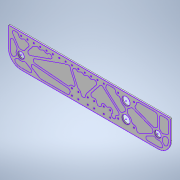
# Autodesk Inventor part: Part2
Saved by Autodesk Inventor 2021 (Build 250183000, 183)
## iProperties
Created: 2020-08-27
Part Number: Part2
Material: Generic
Document SubType Name: Modeling
Designer: gfellows
Density: 1 g/cm^3
Appearance: Default
Author: gfellows
Autodesk Inventor part; units mm, degrees
ref_plane "YZ Plane" through (0, 0, 0) normal (1, 0, 0) x (0, 1, 0)
ref_plane "XZ Plane" through (0, 0, 0) normal (0, 1, 0) x (-1, 0, 0)
ref_plane "XY Plane" through (0, 0, 0) normal (0, 0, 1) x (1, 0, 0)
sketch "Sketch2" plane through (0, 0, 0) normal (0, 0, 1) x (1, 0, 0)
  circle A0 centre (0, 0) radius 50 construction
  circle A1 centre (344, 0) radius 50 construction
  circle A2 centre (264, -8) radius 16 construction
  circle A3 centre (264, 32) radius 16 construction
  circle A4 centre (344, 0) radius 18.8 construction
  circle A5 centre (264, -8) radius 10 construction
  line L0 (261.9218, 1.7817) -> (340.093, 18.3896) construction
  line L1 (263.8999, -17.9995) -> (343.8119, -18.7991) construction
  circle A6 centre (264, 32) radius 10 construction
  circle A7 centre (0, 0) radius 18.8 construction
  line L2 (-1.6434, 18.728) -> (263.1259, 41.9617) construction
  line L3 (2.8786, -18.5783) -> (265.5312, 22.1179) construction
  arc A8 (-32, 0) -> (0, -32) centre (0, 0) ccw
  line L4 (0, -32) -> (344, -32)
  arc A9 (344, -32) -> (376, 0) centre (344, 0) ccw
  line L5 (-32, 0) -> (-32, 50)
  line L6 (-32, 50) -> (376, 50)
  line L7 (376, 50) -> (376, 0)
  circle A10 centre (264, 32) radius 3
  circle A11 centre (264, -8) radius 3
  circle A12 centre (0, 0) radius 8
  circle A13 centre (344, 0) radius 8
  circle A14 centre (264, 32) radius 10
  circle A15 centre (264, -8) radius 10
  circle A16 centre (284, 40) radius 1.5
  circle A17 centre (244, 40) radius 1.5
  circle A18 centre (244, -16) radius 1.5
  circle A19 centre (284, -16) radius 1.5
  circle A20 centre (0, 42) radius 1.5
  circle A21 centre (16, 42) radius 1.5
  circle A22 centre (32, 42) radius 1.5
  circle A23 centre (48, 42) radius 1.5
  circle A24 centre (64, 42) radius 1.5
  circle A25 centre (80, 42) radius 1.5
  circle A26 centre (96, 42) radius 1.5
  circle A27 centre (112, 42) radius 1.5
  circle A28 centre (128, 42) radius 1.5
  circle A29 centre (144, 42) radius 1.5
  circle A30 centre (160, 42) radius 1.5
  circle A31 centre (176, 42) radius 1.5
  circle A32 centre (192, 42) radius 1.5
  circle A33 centre (208, 42) radius 1.5
  circle A34 centre (128, -8) radius 1.5
  circle A35 centre (144, -8) radius 1.5
  circle A36 centre (128, -24) radius 1.5
  circle A37 centre (144, -24) radius 1.5
  circle A38 centre (184, -8) radius 1.5
  circle A39 centre (184, -24) radius 1.5
  circle A40 centre (168, -24) radius 1.5
  circle A41 centre (168, -8) radius 1.5
  circle A42 centre (224, -8) radius 1.5
  circle A43 centre (224, -24) radius 1.5
  circle A44 centre (208, -24) radius 1.5
  circle A45 centre (208, -8) radius 1.5
  dimension "d16" = 100
  dimension "d17" = 100
  dimension "d18" = 32
  dimension "d19" = 32
  dimension "d20" = 20
  dimension "d21" = 20
  dimension "d22" = 37.6
  dimension "d23" = 37.6
  dimension "d25" = 344
  dimension "d26" = 80
  dimension "d27" = 8
  dimension "d28" = 40
  dimension "d29" = 32
  dimension "d30" = 32
  dimension "d31" = 32
  dimension "d32" = 50
  dimension "d33" = 6
  dimension "d34" = 6
  dimension "d35" = 16
  dimension "d36" = 16
  dimension "d37" = 40
  dimension "d38" = 40
  dimension "d39" = 20
  dimension "d40" = 8
  dimension "d41" = 8
  dimension "d42" = 3
  dimension "d43" = 3
  dimension "d44" = 3
  dimension "d45" = 3
  dimension "d48" = 3
  dimension "d49" = 0
  dimension "d50" = 8
  dimension "d53" = 16
  dimension "d59" = 3
  dimension "d60" = 3
  dimension "d61" = 3
  dimension "d62" = 3
  dimension "d63" = 16
  dimension "d64" = 16
  dimension "d65" = 8
  dimension "d66" = 128
  dimension "d69" = 40
  constraints: 46 centre point, 16 end point, 13 coincident, 12 point on circle, 10 tangent, 5 horizontal alignment, 4 vertical alignment, 3 horizontal, 2 concentric, 2 vertical, 1 perpendicular, 42 other
  measures "d16" diameter of A0
  measures "d17" diameter of A1
  measures "d18" diameter of A2
  measures "d19" diameter of A3
  measures "d20" diameter of A6
  measures "d21" diameter of A5
  measures "d22" diameter of A7
  measures "d23" diameter of A4
  measures "d25" distance of A1.centre point (0, 0)
  measures "d26" horizontal distance of A1.centre A2.centre
  measures "d27" vertical distance of A1.centre A2.centre
  measures "d28" distance of A2.centre A3.centre
  measures "d29" distance from line of L5 point (0, 0)
  measures "d30" distance from line of L7 A1.centre
  measures "d31" distance from line of L4 A1.centre
  measures "d32" distance from line of L6 point (0, 0)
  measures "d33" diameter of A10
  measures "d34" diameter of A11
  measures "d35" diameter of A12
  measures "d36" diameter of A13
  measures "d37" distance of A16.centre A17.centre
  measures "d38" distance of A19.centre A18.centre
  measures "d39" horizontal distance of A19.centre A2.centre
  measures "d40" vertical distance of A3.centre A16.centre
  measures "d41" vertical distance of A19.centre A2.centre
  measures "d42" diameter of A17
  measures "d43" diameter of A16
  measures "d44" diameter of A19
  measures "d45" diameter of A18
  measures "d48" diameter of A20
  measures "d49" horizontal distance of A20.centre point (0, 0)
  measures "d50" distance from line of L6 A20.centre
  measures "d53" distance of A20.centre A21.centre
  measures "d59" diameter of A34
  measures "d60" diameter of A35
  measures "d61" diameter of A36
  measures "d62" diameter of A37
  measures "d63" distance of A34.centre A36.centre
  measures "d64" distance of A35.centre A34.centre
  measures "d65" distance from line of L4 A37.centre
  measures "d66" horizontal distance of point (0, 0) A34.centre
  measures "d69" distance of A35.centre A38.centre
extrude "Extrusion1" add sketch "Sketch2" along normal blind 3.175 contours L5 L6 L7 A9 L4 A8
fillet "Fillet1" radius 2 2 edges at (376, 50, 1.5875) (-32, 50, 1.5875)
sketch "Sketch7" plane through (0, 0, 3.175) normal (0, 0, 1) x (1, 0, 0)
  line L0 (374.4783, -9.6992) -> (375.5585, -5.1986)
  line L1 (375.5585, -5.1986) -> (375.6195, -4.8119)
  line L2 (375.6195, -4.8119) -> (375.9901, -0.0994)
  line L3 (375.9901, -0.0994) -> (376.0017, 0.0868)
  line L4 (376.0017, 0.0868) -> (376.0021, 47.8882)
  line L5 (376.0021, 47.8882) -> (375.9918, 48.0939)
  line L6 (375.9918, 48.0939) -> (375.9908, 48.1129)
  line L7 (375.9908, 48.1129) -> (375.9357, 48.4607)
  line L8 (375.9357, 48.4607) -> (375.8388, 48.7576)
  line L9 (375.8388, 48.7576) -> (375.6969, 49.0362)
  line L10 (375.6969, 49.0362) -> (375.514, 49.289)
  line L11 (375.514, 49.289) -> (375.2931, 49.5098)
  line L12 (375.2931, 49.5098) -> (375.0401, 49.6936)
  line L13 (375.0401, 49.6936) -> (374.7621, 49.8354)
  line L14 (374.7621, 49.8354) -> (374.4651, 49.9319)
  line L15 (374.4651, 49.9319) -> (374.1172, 49.987)
  line L16 (374.1172, 49.987) -> (374.0982, 49.9885)
  line L17 (374.0982, 49.9885) -> (373.9022, 49.9962)
  line L18 (373.9022, 49.9962) -> (-29.9016, 49.9999)
  line L19 (-29.9016, 49.9999) -> (-30.0978, 49.9922)
  line L20 (-30.0978, 49.9922) -> (-30.1168, 49.9907)
  line L21 (-30.1168, 49.9907) -> (-30.4647, 49.9356)
  line L22 (-30.4647, 49.9356) -> (-30.7616, 49.8392)
  line L23 (-30.7616, 49.8392) -> (-31.0401, 49.6974)
  line L24 (-31.0401, 49.6974) -> (-31.2929, 49.5138)
  line L25 (-31.2929, 49.5138) -> (-31.5136, 49.293)
  line L26 (-31.5136, 49.293) -> (-31.6972, 49.0402)
  line L27 (-31.6972, 49.0402) -> (-31.839, 48.7617)
  line L28 (-31.839, 48.7617) -> (-31.9355, 48.4648)
  line L29 (-31.9355, 48.4648) -> (-31.9906, 48.117)
  line L30 (-31.9906, 48.117) -> (-31.9921, 48.098)
  line L31 (-31.9921, 48.098) -> (-31.9998, 47.9018)
  line L32 (-31.9998, 47.9018) -> (-32.0002, 0.098)
  line L33 (-32.0002, 0.098) -> (-31.9925, -0.0977)
  line L34 (-31.9925, -0.0977) -> (-31.6216, -4.8101)
  line L35 (-31.6216, -4.8101) -> (-31.5604, -5.1969)
  line L36 (-31.5604, -5.1969) -> (-30.4798, -9.6975)
  line L37 (-30.4798, -9.6975) -> (-30.3588, -10.07)
  line L38 (-30.3588, -10.07) -> (-28.5887, -14.3466)
  line L39 (-28.5887, -14.3466) -> (-28.4108, -14.6956)
  line L40 (-28.4108, -14.6956) -> (-25.9924, -18.642)
  line L41 (-25.9924, -18.642) -> (-25.7621, -18.9589)
  line L42 (-25.7621, -18.9589) -> (-22.7562, -22.4784)
  line L43 (-22.7562, -22.4784) -> (-22.4791, -22.7554)
  line L44 (-22.4791, -22.7554) -> (-18.9589, -25.7604)
  line L45 (-18.9589, -25.7604) -> (-18.642, -25.9907)
  line L46 (-18.642, -25.9907) -> (-14.6957, -28.4092)
  line L47 (-14.6957, -28.4092) -> (-14.3467, -28.587)
  line L48 (-14.3467, -28.587) -> (-10.0704, -30.3582)
  line L49 (-10.0704, -30.3582) -> (-9.698, -30.4792)
  line L50 (-9.698, -30.4792) -> (-5.1972, -31.5594)
  line L51 (-5.1972, -31.5594) -> (-4.8105, -31.6206)
  line L52 (-4.8105, -31.6206) -> (-0.098, -31.9913)
  line L53 (-0.098, -31.9913) -> (0.0977, -31.9989)
  line L54 (0.0977, -31.9989) -> (343.9017, -32.0021)
  line L55 (343.9017, -32.0021) -> (344.0977, -31.9944)
  line L56 (344.0977, -31.9944) -> (348.8097, -31.6235)
  line L57 (348.8097, -31.6235) -> (349.1967, -31.5622)
  line L58 (349.1967, -31.5622) -> (353.6976, -30.4816)
  line L59 (353.6976, -30.4816) -> (354.0696, -30.3606)
  line L60 (354.0696, -30.3606) -> (358.3461, -28.5905)
  line L61 (358.3461, -28.5905) -> (358.6951, -28.4127)
  line L62 (358.6951, -28.4127) -> (362.6419, -25.9939)
  line L63 (362.6419, -25.9939) -> (362.9589, -25.7636)
  line L64 (362.9589, -25.7636) -> (366.4781, -22.758)
  line L65 (366.4781, -22.758) -> (366.755, -22.4809)
  line L66 (366.755, -22.4809) -> (369.7602, -18.9606)
  line L67 (369.7602, -18.9606) -> (369.9901, -18.6437)
  line L68 (369.9901, -18.6437) -> (372.4087, -14.6971)
  line L69 (372.4087, -14.6971) -> (372.5857, -14.3481)
  line L70 (372.5857, -14.3481) -> (374.3573, -10.0717)
  line L71 (374.3573, -10.0717) -> (374.4783, -9.6992)
  line L72 (353.5083, 8.3734) -> (350.2762, 10.7218)
  line L73 (350.2762, 10.7218) -> (348.4596, 13.2222)
  line L74 (348.4596, 13.2222) -> (348.2149, 14.7673)
  line L75 (348.2149, 14.7673) -> (348.2151, 40)
  line L76 (348.2151, 40) -> (349.1701, 42.9389)
  line L77 (349.1701, 42.9389) -> (353.2152, 44.9998)
  line L78 (353.2152, 44.9998) -> (366.0002, 44.9997)
  line L79 (366.0002, 44.9997) -> (368.9391, 44.0447)
  line L80 (368.9391, 44.0447) -> (370.9989, 40.0018)
  line L81 (370.9989, 40.0018) -> (370.9987, 15.8213)
  line L82 (370.9987, 15.8213) -> (370.0438, 12.8824)
  line L83 (370.0438, 12.8824) -> (367.6762, 11.1097)
  line L84 (367.6762, 11.1097) -> (358.1243, 7.7084)
  line L85 (358.1243, 7.7084) -> (355.0353, 7.6221)
  line L86 (355.0353, 7.6221) -> (353.5083, 8.3734)
  line L87 (-2.3107, 12.3636) -> (-5.2496, 13.3185)
  line L88 (-5.2496, 13.3185) -> (-6.5079, 14.6465)
  line L89 (-6.5079, 14.6465) -> (-21.1616, 37.2829)
  line L90 (-21.1616, 37.2829) -> (-21.9571, 40.2689)
  line L91 (-21.9571, 40.2689) -> (-20.8455, 43.1522)
  line L92 (-20.8455, 43.1522) -> (-16.9643, 44.9999)
  line L93 (-16.9643, 44.9999) -> (-11.1074, 44.9999)
  line L94 (-11.1074, 44.9999) -> (-8.1685, 44.0449)
  line L95 (-8.1685, 44.0449) -> (-6.3521, 41.5449)
  line L96 (-6.3521, 41.5449) -> (-5.5034, 38.9323)
  line L97 (-5.5034, 38.9323) -> (-4.618, 37.7137)
  line L98 (-4.618, 37.7137) -> (-2.6494, 36.2833)
  line L99 (-2.6494, 36.2833) -> (-1.2168, 35.8178)
  line L100 (-1.2168, 35.8178) -> (1.2166, 35.8178)
  line L101 (1.2166, 35.8178) -> (2.6492, 36.2832)
  line L102 (2.6492, 36.2832) -> (5.061, 38.0355)
  line L103 (5.061, 38.0355) -> (8, 38.9903)
  line L104 (8, 38.9903) -> (10.9389, 38.0353)
  line L105 (10.9389, 38.0353) -> (13.3507, 36.2829)
  line L106 (13.3507, 36.2829) -> (15.5364, 35.5727)
  line L107 (15.5364, 35.5727) -> (15.5209, 35.5249)
  line L108 (15.5209, 35.5249) -> (17.558, 34.863)
  line L109 (17.558, 34.863) -> (19.3743, 32.363)
  line L110 (19.3743, 32.363) -> (19.3743, 29.2728)
  line L111 (19.3743, 29.2728) -> (18.5549, 27.7343)
  line L112 (18.5549, 27.7343) -> (8.0015, 14.2642)
  line L113 (8.0015, 14.2642) -> (5.4373, 12.5397)
  line L114 (5.4373, 12.5397) -> (4.0171, 12.5655)
  line L115 (4.0171, 12.5655) -> (4.0171, 12.3635)
  line L116 (4.0171, 12.3635) -> (-2.3107, 12.3636)
  line L117 (331.309, 10.0791) -> (331.29, 10.0442)
  line L118 (331.29, 10.0442) -> (331.108, 10.1445)
  line L119 (331.108, 10.1445) -> (331.068, 10.1573)
  line L120 (331.068, 10.1573) -> (331.017, 10.1946)
  line L121 (331.017, 10.1946) -> (330.476, 10.493)
  line L122 (330.476, 10.493) -> (289.462, 26.8484)
  line L123 (289.462, 26.8484) -> (287.086, 28.824)
  line L124 (287.086, 28.824) -> (286.325, 31.819)
  line L125 (286.325, 31.819) -> (288.376, 35.5378)
  line L126 (288.376, 35.5378) -> (288.618, 35.7139)
  line L127 (288.618, 35.7139) -> (289.5033, 36.9323)
  line L128 (289.5033, 36.9323) -> (290.2553, 39.2466)
  line L129 (290.2553, 39.2466) -> (290.2553, 39.9998)
  line L130 (290.2553, 39.9998) -> (291.2102, 42.9387)
  line L131 (291.2102, 42.9387) -> (295.2553, 44.9996)
  line L132 (295.2553, 44.9996) -> (338.2153, 44.9992)
  line L133 (338.2153, 44.9992) -> (341.1543, 44.0442)
  line L134 (341.1543, 44.0442) -> (343.2152, 39.9991)
  line L135 (343.2152, 39.9991) -> (343.215, 16.7886)
  line L136 (343.215, 16.7886) -> (342.2612, 13.8504)
  line L137 (342.2612, 13.8504) -> (339.7612, 12.034)
  line L138 (339.7612, 12.034) -> (339.3422, 11.8981)
  line L139 (339.3422, 11.8981) -> (336.9461, 10.1573)
  line L140 (336.9461, 10.1573) -> (334.007, 9.2025)
  line L141 (334.007, 9.2025) -> (331.309, 10.0791)
  line L142 (247.7696, 2.7223) -> (214.4517, 32.6032)
  line L143 (214.4517, 32.6032) -> (212.901, 35.2763)
  line L144 (212.901, 35.2763) -> (213.499, 38.1013)
  line L145 (213.499, 38.1013) -> (213.259, 38.1794)
  line L146 (213.259, 38.1794) -> (214.3526, 41.5449)
  line L147 (214.3526, 41.5449) -> (216.1692, 44.0452)
  line L148 (216.1692, 44.0452) -> (219.1073, 44.9997)
  line L149 (219.1073, 44.9997) -> (232.7453, 44.9995)
  line L150 (232.7453, 44.9995) -> (235.6843, 44.0446)
  line L151 (235.6843, 44.0446) -> (237.7453, 39.9994)
  line L152 (237.7453, 39.9994) -> (237.7452, 39.2463)
  line L153 (237.7452, 39.2463) -> (238.4971, 36.9319)
  line L154 (238.4971, 36.9319) -> (239.3824, 35.7135)
  line L155 (239.3824, 35.7135) -> (241.3512, 34.2829)
  line L156 (241.3512, 34.2829) -> (242.7832, 33.8176)
  line L157 (242.7832, 33.8176) -> (244.7772, 33.8176)
  line L158 (244.7772, 33.8176) -> (247.7153, 32.8629)
  line L159 (247.7153, 32.8629) -> (249.5319, 30.3626)
  line L160 (249.5319, 30.3626) -> (251.6197, 23.9358)
  line L161 (251.6197, 23.9358) -> (252.505, 22.7173)
  line L162 (252.505, 22.7173) -> (259.3646, 17.7331)
  line L163 (259.3646, 17.7331) -> (259.3596, 17.7292)
  line L164 (259.3596, 17.7292) -> (261.2138, 16.3819)
  line L165 (261.2138, 16.3819) -> (262.1688, 13.4423)
  line L166 (262.1688, 13.4423) -> (262.1688, 10.5493)
  line L167 (262.1688, 10.5493) -> (261.2138, 7.6103)
  line L168 (261.2138, 7.6103) -> (259.3599, 6.2634)
  line L169 (259.3599, 6.2634) -> (259.3602, 6.2608)
  line L170 (259.3602, 6.2608) -> (254.0454, 2.3993)
  line L171 (254.0454, 2.3993) -> (251.1064, 1.4445)
  line L172 (251.1064, 1.4445) -> (247.7696, 2.7223)
  line L173 (17.8113, 12.6027) -> (16.7825, 15.5166)
  line L174 (16.7825, 15.5166) -> (17.845, 18.7263)
  line L175 (17.845, 18.7263) -> (29.7343, 33.9016)
  line L176 (29.7343, 33.9016) -> (32.5598, 35.2774)
  line L177 (32.5598, 35.2774) -> (32.4631, 35.5753)
  line L178 (32.4631, 35.5753) -> (34.6488, 36.2854)
  line L179 (34.6488, 36.2854) -> (37.0606, 38.0376)
  line L180 (37.0606, 38.0376) -> (39.9995, 38.9924)
  line L181 (39.9995, 38.9924) -> (42.9384, 38.0375)
  line L182 (42.9384, 38.0375) -> (45.3502, 36.2851)
  line L183 (45.3502, 36.2851) -> (46.7827, 35.8196)
  line L184 (46.7827, 35.8196) -> (49.2161, 35.8196)
  line L185 (49.2161, 35.8196) -> (50.6488, 36.285)
  line L186 (50.6488, 36.285) -> (53.0606, 38.0373)
  line L187 (53.0606, 38.0373) -> (55.9995, 38.992)
  line L188 (55.9995, 38.992) -> (58.9384, 38.0371)
  line L189 (58.9384, 38.0371) -> (61.3502, 36.2847)
  line L190 (61.3502, 36.2847) -> (62.7827, 35.8192)
  line L191 (62.7827, 35.8192) -> (64.7633, 35.8192)
  line L192 (64.7633, 35.8192) -> (66.1505, 35.3685)
  line L193 (66.1505, 35.3685) -> (66.227, 35.6258)
  line L194 (66.227, 35.6258) -> (67.406, 36.8349)
  line L195 (67.406, 36.8349) -> (69.0605, 38.037)
  line L196 (69.0605, 38.037) -> (71.9995, 38.9917)
  line L197 (71.9995, 38.9917) -> (74.9384, 38.0368)
  line L198 (74.9384, 38.0368) -> (75.5107, 37.6209)
  line L199 (75.5107, 37.6209) -> (77.3273, 35.1206)
  line L200 (77.3273, 35.1206) -> (77.3273, 32.0304)
  line L201 (77.3273, 32.0304) -> (74.2367, 28.8607)
  line L202 (74.2367, 28.8607) -> (72.0099, 28.0745)
  line L203 (72.0099, 28.0745) -> (68.9207, 27.9965)
  line L204 (68.9207, 27.9965) -> (68.5337, 28.263)
  line L205 (68.5337, 28.263) -> (66.4283, 26.1038)
  line L206 (66.4283, 26.1038) -> (23.4455, 10.928)
  line L207 (23.4455, 10.928) -> (20.3563, 10.85)
  line L208 (20.3563, 10.85) -> (17.8113, 12.6027)
  line L209 (155.2548, -13.6224) -> (152.3158, -12.6675)
  line L210 (152.3158, -12.6675) -> (150.2549, -8.6224)
  line L211 (150.2549, -8.6224) -> (150.255, -7.2468)
  line L212 (150.255, -7.2468) -> (149.5031, -4.9325)
  line L213 (149.5031, -4.9325) -> (148.6179, -3.7141)
  line L214 (148.6179, -3.7141) -> (146.649, -2.2835)
  line L215 (146.649, -2.2835) -> (145.592, -1.9401)
  line L216 (145.592, -1.9401) -> (142.543, 0.8412)
  line L217 (142.543, 0.8412) -> (129.684, 30.7658)
  line L218 (129.684, 30.7658) -> (129.401, 33.843)
  line L219 (129.401, 33.843) -> (131.339, 36.7849)
  line L220 (131.339, 36.7849) -> (133.0609, 38.036)
  line L221 (133.0609, 38.036) -> (136, 38.9908)
  line L222 (136, 38.9908) -> (138.939, 38.0358)
  line L223 (138.939, 38.0358) -> (141.3509, 36.2833)
  line L224 (141.3509, 36.2833) -> (142.7829, 35.818)
  line L225 (142.7829, 35.818) -> (145.2169, 35.818)
  line L226 (145.2169, 35.818) -> (146.649, 36.2832)
  line L227 (146.649, 36.2832) -> (149.0609, 38.0356)
  line L228 (149.0609, 38.0356) -> (152, 38.9904)
  line L229 (152, 38.9904) -> (154.939, 38.0354)
  line L230 (154.939, 38.0354) -> (157.3508, 36.283)
  line L231 (157.3508, 36.283) -> (158.7829, 35.8177)
  line L232 (158.7829, 35.8177) -> (161.2169, 35.8176)
  line L233 (161.2169, 35.8176) -> (162.649, 36.2829)
  line L234 (162.649, 36.2829) -> (165.0609, 38.0352)
  line L235 (165.0609, 38.0352) -> (168, 38.99)
  line L236 (168, 38.99) -> (170.939, 38.0351)
  line L237 (170.939, 38.0351) -> (173.3508, 36.2826)
  line L238 (173.3508, 36.2826) -> (174.7829, 35.8173)
  line L239 (174.7829, 35.8173) -> (177.2169, 35.8173)
  line L240 (177.2169, 35.8173) -> (178.649, 36.2825)
  line L241 (178.649, 36.2825) -> (181.0609, 38.0349)
  line L242 (181.0609, 38.0349) -> (184, 38.9897)
  line L243 (184, 38.9897) -> (186.9389, 38.0347)
  line L244 (186.9389, 38.0347) -> (188.324, 37.0283)
  line L245 (188.324, 37.0283) -> (190.1406, 34.528)
  line L246 (190.1406, 34.528) -> (190.1406, 31.4378)
  line L247 (190.1406, 31.4378) -> (189.2972, 29.861)
  line L248 (189.2972, 29.861) -> (164.7591, -0.8634)
  line L249 (164.7591, -0.8634) -> (164.338, -1.6443)
  line L250 (164.338, -1.6443) -> (164.1399, -2.2549)
  line L251 (164.1399, -2.2549) -> (163.4297, -3.6487)
  line L252 (163.4297, -3.6487) -> (162.4968, -4.9327)
  line L253 (162.4968, -4.9327) -> (161.7448, -7.247)
  line L254 (161.7448, -7.247) -> (161.7448, -8.6225)
  line L255 (161.7448, -8.6225) -> (160.7899, -11.5614)
  line L256 (160.7899, -11.5614) -> (158.2898, -13.3777)
  line L257 (158.2898, -13.3777) -> (156.7448, -13.6224)
  line L258 (156.7448, -13.6224) -> (155.2548, -13.6224)
  line L259 (34.6019, -0.5648) -> (31.7567, 0.6412)
  line L260 (31.7567, 0.6412) -> (30.1637, 3.2891)
  line L261 (30.1637, 3.2891) -> (30.4315, 6.3677)
  line L262 (30.4315, 6.3677) -> (33.3706, 9.131)
  line L263 (33.3706, 9.131) -> (104.1632, 34.1255)
  line L264 (104.1632, 34.1255) -> (104.7972, 34.4586)
  line L265 (104.7972, 34.4586) -> (105.7552, 35.1541)
  line L266 (105.7552, 35.1541) -> (105.8754, 34.9886)
  line L267 (105.8754, 34.9886) -> (107.2256, 35.9695)
  line L268 (107.2256, 35.9695) -> (110.3166, 35.9695)
  line L269 (110.3166, 35.9695) -> (110.7836, 35.8175)
  line L270 (110.7836, 35.8175) -> (113.2176, 35.8175)
  line L271 (113.2176, 35.8175) -> (114.6497, 36.2828)
  line L272 (114.6497, 36.2828) -> (116.3065, 37.4865)
  line L273 (116.3065, 37.4865) -> (119.2455, 38.4413)
  line L274 (119.2455, 38.4413) -> (122.1845, 37.4863)
  line L275 (122.1845, 37.4863) -> (124.2454, 33.4412)
  line L276 (124.2454, 33.4412) -> (124.2454, 31.2461)
  line L277 (124.2454, 31.2461) -> (124.4423, 30.6389)
  line L278 (124.4423, 30.6389) -> (124.5233, 30.4242)
  line L279 (124.5233, 30.4242) -> (135.5081, 4.8609)
  line L280 (135.5081, 4.8609) -> (135.7911, 1.7846)
  line L281 (135.7911, 1.7846) -> (134.2113, -0.8714)
  line L282 (134.2113, -0.8714) -> (131.3723, -2.0914)
  line L283 (131.3723, -2.0914) -> (129.3693, -1.8677)
  line L284 (129.3693, -1.8677) -> (129.2173, -1.8183)
  line L285 (129.2173, -1.8183) -> (126.7833, -1.8182)
  line L286 (126.7833, -1.8182) -> (125.3513, -2.2835)
  line L287 (125.3513, -2.2835) -> (123.3824, -3.7139)
  line L288 (123.3824, -3.7139) -> (122.0295, -5.5759)
  line L289 (122.0295, -5.5759) -> (121.8738, -5.4628)
  line L290 (121.8738, -5.4628) -> (120.8734, -6.8396)
  line L291 (120.8734, -6.8396) -> (117.5014, -7.7756)
  line L292 (117.5014, -7.7756) -> (34.6019, -0.5648)
  line L293 (228.6909, -19.8299) -> (228.1429, -19.0767)
  line L294 (228.1429, -19.0767) -> (228.2839, -18.9744)
  line L295 (228.2839, -18.9744) -> (227.248, -17.5486)
  line L296 (227.248, -17.5486) -> (227.2481, -14.4584)
  line L297 (227.2481, -14.4584) -> (228.2841, -13.0325)
  line L298 (228.2841, -13.0325) -> (228.1431, -12.9302)
  line L299 (228.1431, -12.9302) -> (228.6912, -12.1771)
  line L300 (228.6912, -12.1771) -> (230.8133, -10.6353)
  line L301 (230.8133, -10.6353) -> (230.2466, -8.891)
  line L302 (230.2466, -8.891) -> (230.2467, -7.2504)
  line L303 (230.2467, -7.2504) -> (229.4948, -4.936)
  line L304 (229.4948, -4.936) -> (228.6096, -3.7176)
  line L305 (228.6096, -3.7176) -> (226.6407, -2.2871)
  line L306 (226.6407, -2.2871) -> (225.2087, -1.8217)
  line L307 (225.2087, -1.8217) -> (222.7747, -1.8217)
  line L308 (222.7747, -1.8217) -> (221.3426, -2.2869)
  line L309 (221.3426, -2.2869) -> (218.9307, -4.0393)
  line L310 (218.9307, -4.0393) -> (215.9916, -4.9941)
  line L311 (215.9916, -4.9941) -> (213.0526, -4.0391)
  line L312 (213.0526, -4.0391) -> (210.6408, -2.2867)
  line L313 (210.6408, -2.2867) -> (209.2087, -1.8214)
  line L314 (209.2087, -1.8214) -> (206.7747, -1.8214)
  line L315 (206.7747, -1.8214) -> (205.3426, -2.2866)
  line L316 (205.3426, -2.2866) -> (203.3738, -3.7171)
  line L317 (203.3738, -3.7171) -> (202.4885, -4.9355)
  line L318 (202.4885, -4.9355) -> (201.7365, -7.2498)
  line L319 (201.7365, -7.2498) -> (201.7365, -8.6253)
  line L320 (201.7365, -8.6253) -> (200.7815, -11.5642)
  line L321 (200.7815, -11.5642) -> (198.2815, -13.3805)
  line L322 (198.2815, -13.3805) -> (196.7365, -13.6252)
  line L323 (196.7365, -13.6252) -> (195.2465, -13.6252)
  line L324 (195.2465, -13.6252) -> (192.3075, -12.6703)
  line L325 (192.3075, -12.6703) -> (190.2466, -8.6252)
  line L326 (190.2466, -8.6252) -> (190.2466, -7.2496)
  line L327 (190.2466, -7.2496) -> (189.4948, -4.9353)
  line L328 (189.4948, -4.9353) -> (188.6095, -3.7169)
  line L329 (188.6095, -3.7169) -> (186.6407, -2.2863)
  line L330 (186.6407, -2.2863) -> (185.2087, -1.821)
  line L331 (185.2087, -1.821) -> (182.7747, -1.821)
  line L332 (182.7747, -1.821) -> (181.8897, -2.1085)
  line L333 (181.8897, -2.1085) -> (178.7997, -2.1085)
  line L334 (178.7997, -2.1085) -> (176.2997, -0.292)
  line L335 (176.2997, -0.292) -> (175.3449, 2.647)
  line L336 (175.3449, 2.647) -> (176.4382, 5.7666)
  line L337 (176.4382, 5.7666) -> (198.4957, 33.3851)
  line L338 (198.4957, 33.3851) -> (201.0759, 35.0857)
  line L339 (201.0759, 35.0857) -> (204.1629, 34.9448)
  line L340 (204.1629, 34.9448) -> (205.9007, 33.5484)
  line L341 (205.9007, 33.5484) -> (205.9727, 33.6296)
  line L342 (205.9727, 33.6296) -> (244.8683, -1.2536)
  line L343 (244.8683, -1.2536) -> (246.419, -3.9267)
  line L344 (246.419, -3.9267) -> (246.1032, -6.9928)
  line L345 (246.1032, -6.9928) -> (243.0761, -9.7238)
  line L346 (243.0761, -9.7238) -> (241.342, -10.2871)
  line L347 (241.342, -10.2871) -> (239.3732, -11.7176)
  line L348 (239.3732, -11.7176) -> (239.2912, -11.8301)
  line L349 (239.2912, -11.8301) -> (237.1691, -13.3719)
  line L350 (237.1691, -13.3719) -> (237.7357, -15.1162)
  line L351 (237.7357, -15.1162) -> (237.7357, -16.8911)
  line L352 (237.7357, -16.8911) -> (236.7808, -19.83)
  line L353 (236.7808, -19.83) -> (234.2808, -21.6464)
  line L354 (234.2808, -21.6464) -> (231.1908, -21.6464)
  line L355 (231.1908, -21.6464) -> (228.6909, -19.8299)
  line L356 (-23.26, -11.7395) -> (-25.216, -9.4204)
  line L357 (-25.216, -9.4204) -> (-25.5133, -8.7021)
  line L358 (-25.5133, -8.7021) -> (-25.7557, -7.956)
  line L359 (-25.7557, -7.956) -> (-26.5605, -4.604)
  line L360 (-26.5605, -4.604) -> (-26.6832, -3.8291)
  line L361 (-26.6832, -3.8291) -> (-26.9847, 0.0007)
  line L362 (-26.9847, 0.0007) -> (-27.0001, 0.393)
  line L363 (-27.0001, 0.393) -> (-26.9999, 20.1896)
  line L364 (-26.9999, 20.1896) -> (-26.045, 23.1285)
  line L365 (-26.045, 23.1285) -> (-23.545, 24.9449)
  line L366 (-23.545, 24.9449) -> (-20.4548, 24.9448)
  line L367 (-20.4548, 24.9448) -> (-17.8026, 22.9066)
  line L368 (-17.8026, 22.9066) -> (-10.866, 12.1912)
  line L369 (-10.866, 12.1912) -> (-10.0705, 9.2052)
  line L370 (-10.0705, 9.2052) -> (-10.6145, 7.6727)
  line L371 (-10.6145, 7.6727) -> (-10.5154, 7.6404)
  line L372 (-10.5154, 7.6404) -> (-12.7544, 0.7496)
  line L373 (-12.7544, 0.7496) -> (-12.7544, -0.7567)
  line L374 (-12.7544, -0.7567) -> (-12.0806, -2.8307)
  line L375 (-12.0806, -2.8307) -> (-12.0807, -5.9209)
  line L376 (-12.0807, -5.9209) -> (-13.6347, -8.2157)
  line L377 (-13.6347, -8.2157) -> (-17.3951, -11.3494)
  line L378 (-17.3951, -11.3494) -> (-20.2642, -12.4973)
  line L379 (-20.2642, -12.4973) -> (-23.26, -11.7395)
  line L380 (291.6642, -20.353) -> (290.2542, -16.8733)
  line L381 (290.2542, -16.8733) -> (290.2542, -15.2472)
  line L382 (290.2542, -15.2472) -> (289.5024, -12.9328)
  line L383 (289.5024, -12.9328) -> (288.6171, -11.7144)
  line L384 (288.6171, -11.7144) -> (286.6483, -10.2838)
  line L385 (286.6483, -10.2838) -> (285.2163, -9.8185)
  line L386 (285.2163, -9.8185) -> (283.2223, -9.8185)
  line L387 (283.2223, -9.8185) -> (280.2842, -8.8638)
  line L388 (280.2842, -8.8638) -> (278.4676, -6.3635)
  line L389 (278.4676, -6.3635) -> (276.3798, 0.0633)
  line L390 (276.3798, 0.0633) -> (275.4945, 1.2818)
  line L391 (275.4945, 1.2818) -> (269.2329, 5.8314)
  line L392 (269.2329, 5.8314) -> (267.4167, 8.3313)
  line L393 (267.4167, 8.3313) -> (267.172, 9.8764)
  line L394 (267.172, 9.8764) -> (267.172, 14.1236)
  line L395 (267.172, 14.1236) -> (268.127, 17.0625)
  line L396 (268.127, 17.0625) -> (269.2328, 18.1689)
  line L397 (269.2328, 18.1689) -> (275.4945, 22.7183)
  line L398 (275.4945, 22.7183) -> (275.6475, 22.9294)
  line L399 (275.6475, 22.9294) -> (278.1475, 24.7458)
  line L400 (278.1475, 24.7458) -> (281.5445, 24.6347)
  line L401 (281.5445, 24.6347) -> (328.0966, 6.0709)
  line L402 (328.0966, 6.0709) -> (330.4726, 4.0953)
  line L403 (330.4726, 4.0953) -> (331.2446, 1.4265)
  line L404 (331.2446, 1.4265) -> (331.2446, -1.5458)
  line L405 (331.2446, -1.5458) -> (331.0404, -1.5458)
  line L406 (331.0404, -1.5458) -> (331.0403, -3.2159)
  line L407 (331.0403, -3.2159) -> (328.4843, -6.1608)
  line L408 (328.4843, -6.1608) -> (297.4542, -21.3634)
  line L409 (297.4542, -21.3634) -> (294.3952, -21.7989)
  line L410 (294.3952, -21.7989) -> (291.6642, -20.353)
  line L411 (359.132, -14.5813) -> (356.029, -11.192)
  line L412 (356.029, -11.192) -> (354.749, -8.3794)
  line L413 (354.749, -8.3794) -> (354.962, -6.271)
  line L414 (354.962, -6.271) -> (356.975, -0.0757)
  line L415 (356.975, -0.0757) -> (360.0541, 3.0895)
  line L416 (360.0541, 3.0895) -> (364.283, 4.5954)
  line L417 (364.283, 4.5954) -> (367.372, 4.6817)
  line L418 (367.372, 4.6817) -> (369.9221, 2.9359)
  line L419 (369.9221, 2.9359) -> (370.9453, -0.5069)
  line L420 (370.9453, -0.5069) -> (370.6834, -3.829)
  line L421 (370.6834, -3.829) -> (370.5603, -4.6039)
  line L422 (370.5603, -4.6039) -> (369.7559, -7.9558)
  line L423 (369.7559, -7.9558) -> (369.5128, -8.7019)
  line L424 (369.5128, -8.7019) -> (368.1937, -11.8869)
  line L425 (368.1937, -11.8869) -> (367.8377, -12.586)
  line L426 (367.8377, -12.586) -> (367.0829, -13.8177)
  line L427 (367.0829, -13.8177) -> (364.733, -15.8247)
  line L428 (364.733, -15.8247) -> (361.653, -16.0672)
  line L429 (361.653, -16.0672) -> (359.132, -14.5813)
  line L430 (49.5735, -27.0002) -> (46.6346, -26.0453)
  line L431 (46.6346, -26.0453) -> (45.7411, -25.3961)
  line L432 (45.7411, -25.3961) -> (45.5849, -25.2914)
  line L433 (45.5849, -25.2914) -> (27.9029, -14.3736)
  line L434 (27.9029, -14.3736) -> (25.9039, -12.0171)
  line L435 (25.9039, -12.0171) -> (25.6718, -8.9357)
  line L436 (25.6718, -8.9357) -> (27.2953, -6.3063)
  line L437 (27.2953, -6.3063) -> (30.963, -5.138)
  line L438 (30.963, -5.138) -> (119.04, -12.7991)
  line L439 (119.04, -12.7991) -> (121.885, -14.0051)
  line L440 (121.885, -14.0051) -> (123.478, -16.653)
  line L441 (123.478, -16.653) -> (122.6516, -20.7201)
  line L442 (122.6516, -20.7201) -> (122.4966, -20.9335)
  line L443 (122.4966, -20.9335) -> (121.6477, -23.5461)
  line L444 (121.6477, -23.5461) -> (119.831, -26.0463)
  line L445 (119.831, -26.0463) -> (116.8929, -27.0008)
  line L446 (116.8929, -27.0008) -> (49.5735, -27.0002)
  line L447 (318.7702, -26.9999) -> (315.8312, -26.0449)
  line L448 (315.8312, -26.0449) -> (314.015, -23.5451)
  line L449 (314.015, -23.5451) -> (314.015, -20.4549)
  line L450 (314.015, -20.4549) -> (316.57, -17.5099)
  line L451 (316.57, -17.5099) -> (332.0801, -9.9111)
  line L452 (332.0801, -9.9111) -> (335.1401, -9.4755)
  line L453 (335.1401, -9.4755) -> (337.2191, -10.3559)
  line L454 (337.2191, -10.3559) -> (339.342, -11.8984)
  line L455 (339.342, -11.8984) -> (340.775, -12.364)
  line L456 (340.775, -12.364) -> (348.0185, -12.3641)
  line L457 (348.0185, -12.3641) -> (348.0185, -12.5721)
  line L458 (348.0185, -12.5721) -> (349.6772, -12.5721)
  line L459 (349.6772, -12.5721) -> (351.8202, -13.9516)
  line L460 (351.8202, -13.9516) -> (354.9182, -17.3363)
  line L461 (354.9182, -17.3363) -> (356.1982, -20.149)
  line L462 (356.1982, -20.149) -> (355.5807, -23.1767)
  line L463 (355.5807, -23.1767) -> (353.1433, -25.331)
  line L464 (353.1433, -25.331) -> (352.7022, -25.5133)
  line L465 (352.7022, -25.5133) -> (351.9562, -25.7557)
  line L466 (351.9562, -25.7557) -> (348.6042, -26.5605)
  line L467 (348.6042, -26.5605) -> (347.8292, -26.6832)
  line L468 (347.8292, -26.6832) -> (343.9992, -26.9847)
  line L469 (343.9992, -26.9847) -> (343.6072, -27.0001)
  line L470 (343.6072, -27.0001) -> (318.7702, -26.9999)
  line L471 (0.3931, -26.9995) -> (0.0007, -26.9841)
  line L472 (0.0007, -26.9841) -> (-3.829, -26.6829)
  line L473 (-3.829, -26.6829) -> (-4.604, -26.5601)
  line L474 (-4.604, -26.5601) -> (-7.956, -25.7557)
  line L475 (-7.956, -25.7557) -> (-8.7022, -25.5132)
  line L476 (-8.7022, -25.5132) -> (-11.8872, -24.194)
  line L477 (-11.8872, -24.194) -> (-12.5863, -23.8378)
  line L478 (-12.5863, -23.8378) -> (-13.6874, -23.163)
  line L479 (-13.6874, -23.163) -> (-15.6943, -20.8132)
  line L480 (-15.6943, -20.8132) -> (-15.9368, -17.7326)
  line L481 (-15.9368, -17.7326) -> (-14.2769, -15.0595)
  line L482 (-14.2769, -15.0595) -> (-10.7618, -12.1303)
  line L483 (-10.7618, -12.1303) -> (-7.8927, -10.9824)
  line L484 (-7.8927, -10.9824) -> (-5.4231, -11.6954)
  line L485 (-5.4231, -11.6954) -> (-5.4099, -11.6548)
  line L486 (-5.4099, -11.6548) -> (-3.225, -12.3648)
  line L487 (-3.225, -12.3648) -> (3.2256, -12.3648)
  line L488 (3.2256, -12.3648) -> (4.6581, -11.8994)
  line L489 (4.6581, -11.8994) -> (6.5346, -10.5361)
  line L490 (6.5346, -10.5361) -> (9.4736, -9.5814)
  line L491 (9.4736, -9.5814) -> (12.1003, -10.327)
  line L492 (12.1003, -10.327) -> (24.1177, -17.7471)
  line L493 (24.1177, -17.7471) -> (26.1167, -20.1036)
  line L494 (26.1167, -20.1036) -> (26.3486, -23.1833)
  line L495 (26.3486, -23.1833) -> (24.7252, -25.8126)
  line L496 (24.7252, -25.8126) -> (21.4907, -26.9997)
  line L497 (21.4907, -26.9997) -> (0.3931, -26.9995)
  circle A0 centre (208, -8) radius 1.5
  circle A1 centre (224, -24) radius 1.5
  circle A2 centre (168, -8) radius 1.5
  circle A3 centre (184, -24) radius 1.5
  circle A4 centre (144, -24) radius 1.5
  circle A5 centre (144, -8) radius 1.5
  circle A6 centre (208, 42) radius 1.5
  circle A7 centre (176, 42) radius 1.5
  circle A8 centre (144, 42) radius 1.5
  circle A9 centre (112, 42) radius 1.5
  circle A10 centre (80, 42) radius 1.5
  circle A11 centre (48, 42) radius 1.5
  circle A12 centre (32, 42) radius 1.5
  circle A13 centre (16, 42) radius 1.5
  circle A14 centre (0, 42) radius 1.5
  circle A15 centre (284, -16) radius 1.5
  circle A16 centre (244, -16) radius 1.5
  circle A17 centre (244, 40) radius 1.5
  circle A18 centre (284, 40) radius 1.5
  circle A19 centre (64, 42) radius 1.5
  circle A20 centre (96, 42) radius 1.5
  circle A21 centre (128, 42) radius 1.5
  circle A22 centre (160, 42) radius 1.5
  circle A23 centre (192, 42) radius 1.5
  circle A24 centre (128, -8) radius 1.5
  circle A25 centre (128, -24) radius 1.5
  circle A26 centre (184, -8) radius 1.5
  circle A27 centre (168, -24) radius 1.5
  circle A28 centre (224, -8) radius 1.5
  circle A29 centre (208, -24) radius 1.5
  circle A30 centre (264, -8) radius 10
  circle A31 centre (264, 32) radius 10
  circle A32 centre (344, 0) radius 8
  circle A33 centre (0, 0) radius 8
  constraints: 996 end point, 225 parallel, 125 perpendicular, 34 centre point, 31 equal radius
sketch "Sketch8" plane through (0, 0, 3.175) normal (0, 0, 1) x (1, 0, 0)
  point P0 (0, 0)
equation "\"d21\" = d20"
equation "\"d32\" = 0.5 * d16"
body "Solid1"
